Autodesk Inventor part; units mm, degrees
(part 3 of 5)
  line L1368 (280.713, 47.7132) -> (279.888, 47.7132) projected
  line L1369 (280.713, 50.3135) -> (280.713, 47.7132) projected
  line L1370 (279.888, 50.3135) -> (280.713, 50.3135) projected
  line L1371 (279.888, 53.5421) -> (279.888, 50.3135) projected
  line L1372 (273.338, 53.5421) -> (279.888, 53.5421) projected
  line L1373 (273.338, 50.3135) -> (273.338, 53.5421) projected
  line L1374 (271.614, 50.3135) -> (273.338, 50.3135) projected
  line L1375 (271.614, 55.0125) -> (271.614, 50.3135) projected
  line L1376 (226.858, 41.2129) -> (226.858, 55.0125) projected
  line L1377 (240.658, 41.2129) -> (226.858, 41.2129) projected
  line L1378 (240.658, 55.0125) -> (240.658, 41.2129) projected
  line L1379 (226.858, 55.0125) -> (240.658, 55.0125) projected
  line L1380 (221.608, 55.0125) -> (221.608, 41.2129) projected
  line L1381 (207.808, 55.0125) -> (221.608, 55.0125) projected
  line L1382 (207.808, 41.2129) -> (207.808, 55.0125) projected
  line L1383 (221.608, 41.2129) -> (207.808, 41.2129) projected
  line L1384 (202.558, 41.2129) -> (188.758, 41.2129) projected
  line L1385 (202.558, 55.0125) -> (202.558, 41.2129) projected
  line L1386 (188.758, 55.0125) -> (202.558, 55.0125) projected
  line L1387 (188.758, 41.2129) -> (188.758, 55.0125) projected
  line L1388 (122.083, 35.9625) -> (135.883, 35.9625) projected
  line L1389 (122.083, 22.163) -> (122.083, 35.9625) projected
  line L1390 (135.883, 22.163) -> (122.083, 22.163) projected
  line L1391 (135.883, 35.9625) -> (135.883, 22.163) projected
  line L1392 (195.902, 16.9127) -> (209.702, 16.9127) projected
  line L1393 (195.902, 3.113) -> (195.902, 16.9127) projected
  line L1394 (209.702, 3.113) -> (195.902, 3.113) projected
  line L1395 (209.702, 16.9127) -> (209.702, 3.113) projected
  line L1396 (193.033, 22.163) -> (179.233, 22.163) projected
  line L1397 (193.033, 35.9625) -> (193.033, 22.163) projected
  line L1398 (179.233, 35.9625) -> (193.033, 35.9625) projected
  line L1399 (179.233, 22.163) -> (179.233, 35.9625) projected
  line L1400 (160.183, 22.163) -> (160.183, 35.9625) projected
  line L1401 (173.983, 22.163) -> (160.183, 22.163) projected
  line L1402 (173.983, 35.9625) -> (173.983, 22.163) projected
  line L1403 (160.183, 35.9625) -> (173.983, 35.9625) projected
  line L1404 (141.133, 22.163) -> (141.133, 35.9625) projected
  line L1405 (154.933, 22.163) -> (141.133, 22.163) projected
  line L1406 (154.933, 35.9625) -> (154.933, 22.163) projected
  line L1407 (141.133, 35.9625) -> (154.933, 35.9625) projected
  line L1408 (73.9704, 103.125) -> (60.1694, 103.125) projected
  line L1409 (73.9704, 116.926) -> (73.9704, 103.125) projected
  line L1410 (60.1694, 116.926) -> (73.9704, 116.926) projected
  line L1411 (60.1694, 103.125) -> (60.1694, 116.926) projected
  line L1412 (131.12, 79.3129) -> (117.321, 79.3129) projected
  line L1413 (131.12, 93.1125) -> (131.12, 79.3129) projected
  line L1414 (117.321, 93.1125) -> (131.12, 93.1125) projected
  line L1415 (117.321, 79.3129) -> (117.321, 93.1125) projected
  line L1416 (112.07, 79.3129) -> (98.2694, 79.3129) projected
  line L1417 (112.07, 93.1125) -> (112.07, 79.3129) projected
  line L1418 (98.2694, 93.1125) -> (112.07, 93.1125) projected
  line L1419 (98.2694, 79.3129) -> (98.2694, 93.1125) projected
  line L1420 (140.645, 74.0625) -> (140.645, 60.2629) projected
  line L1421 (126.846, 74.0625) -> (140.645, 74.0625) projected
  line L1422 (126.846, 60.2629) -> (126.846, 74.0625) projected
  line L1423 (140.645, 60.2629) -> (126.846, 60.2629) projected
  line L1424 (145.896, 74.0625) -> (159.695, 74.0625) projected
  line L1425 (145.896, 60.2629) -> (145.896, 74.0625) projected
  line L1426 (159.695, 60.2629) -> (145.896, 60.2629) projected
  line L1427 (159.695, 74.0625) -> (159.695, 60.2629) projected
  line L1428 (93.0204, 103.125) -> (79.2194, 103.125) projected
  line L1429 (93.0204, 116.926) -> (93.0204, 103.125) projected
  line L1430 (79.2194, 116.926) -> (93.0204, 116.926) projected
  line L1431 (79.2194, 103.125) -> (79.2194, 116.926) projected
  line L1432 (112.558, 41.2129) -> (112.558, 55.0125) projected
  line L1433 (126.358, 41.2129) -> (112.558, 41.2129) projected
  line L1434 (126.358, 55.0125) -> (126.358, 41.2129) projected
  line L1435 (112.558, 55.0125) -> (126.358, 55.0125) projected
  line L1436 (54.919, 103.125) -> (41.1208, 103.125) projected
  line L1437 (54.919, 116.926) -> (54.919, 103.125) projected
  line L1438 (41.1208, 116.926) -> (54.919, 116.926) projected
  line L1439 (41.1208, 103.125) -> (41.1208, 116.926) projected
  line L1440 (102.545, 74.0625) -> (102.545, 60.2629) projected
  line L1441 (88.7444, 74.0625) -> (102.545, 74.0625) projected
  line L1442 (88.7444, 60.2629) -> (88.7444, 74.0625) projected
  line L1443 (102.545, 60.2629) -> (88.7444, 60.2629) projected
  line L1444 (107.794, 60.2629) -> (107.794, 74.0625) projected
  line L1445 (121.595, 60.2629) -> (107.794, 60.2629) projected
  line L1446 (121.595, 74.0625) -> (121.595, 60.2629) projected
  line L1447 (107.794, 74.0625) -> (121.595, 74.0625) projected
  line L1448 (79.2194, 79.3129) -> (79.2194, 93.1125) projected
  line L1449 (93.0204, 79.3129) -> (79.2194, 79.3129) projected
  line L1450 (93.0204, 93.1125) -> (93.0204, 79.3129) projected
  line L1451 (79.2194, 93.1125) -> (93.0204, 93.1125) projected
  line L1452 (73.9704, 79.3129) -> (60.1694, 79.3129) projected
  line L1453 (73.9704, 93.1125) -> (73.9704, 79.3129) projected
  line L1454 (60.1694, 93.1125) -> (73.9704, 93.1125) projected
  line L1455 (60.1694, 79.3129) -> (60.1694, 93.1125) projected
  line L1456 (50.6458, 74.0625) -> (64.4454, 74.0625) projected
  line L1457 (50.6458, 60.2629) -> (50.6458, 74.0625) projected
  line L1458 (64.4454, 60.2629) -> (50.6458, 60.2629) projected
  line L1459 (64.4454, 74.0625) -> (64.4454, 60.2629) projected
  line L1460 (83.4954, 60.2629) -> (69.6958, 60.2629) projected
  line L1461 (83.4954, 74.0625) -> (83.4954, 60.2629) projected
  line L1462 (69.6958, 74.0625) -> (83.4954, 74.0625) projected
  line L1463 (69.6958, 60.2629) -> (69.6958, 74.0625) projected
  line L1464 (74.4583, 41.2129) -> (74.4583, 55.0125) projected
  line L1465 (88.2579, 41.2129) -> (74.4583, 41.2129) projected
  line L1466 (88.2579, 55.0125) -> (88.2579, 41.2129) projected
  line L1467 (74.4583, 55.0125) -> (88.2579, 55.0125) projected
  line L1468 (41.1208, 79.3129) -> (41.1208, 93.1125) projected
  line L1469 (54.919, 79.3129) -> (41.1208, 79.3129) projected
  line L1470 (54.919, 93.1125) -> (54.919, 79.3129) projected
  line L1471 (41.1208, 93.1125) -> (54.919, 93.1125) projected
  line L1472 (107.308, 41.2129) -> (93.5083, 41.2129) projected
  line L1473 (107.308, 55.0125) -> (107.308, 41.2129) projected
  line L1474 (93.5083, 55.0125) -> (107.308, 55.0125) projected
  line L1475 (93.5083, 41.2129) -> (93.5083, 55.0125) projected
  line L1476 (103.033, 22.163) -> (103.033, 35.9625) projected
  line L1477 (116.833, 22.163) -> (103.033, 22.163) projected
  line L1478 (116.833, 35.9625) -> (116.833, 22.163) projected
  line L1479 (103.033, 35.9625) -> (116.833, 35.9625) projected
  line L1480 (97.7829, 35.9625) -> (97.7829, 22.163) projected
  line L1481 (83.9833, 35.9625) -> (97.7829, 35.9625) projected
  line L1482 (83.9833, 22.163) -> (83.9833, 35.9625) projected
  line L1483 (97.7829, 22.163) -> (83.9833, 22.163) projected
  line L1484 (16.8203, 103.125) -> (3.0193, 103.125) projected
  line L1485 (16.8203, 116.926) -> (16.8203, 103.125) projected
  line L1486 (3.0193, 116.926) -> (16.8203, 116.926) projected
  line L1487 (3.0193, 103.125) -> (3.0193, 116.926) projected
  line L1488 (16.8203, 79.3129) -> (3.0193, 79.3129) projected
  line L1489 (16.8203, 93.1125) -> (16.8203, 79.3129) projected
  line L1490 (3.0193, 93.1125) -> (16.8203, 93.1125) projected
  line L1491 (3.0193, 79.3129) -> (3.0193, 93.1125) projected
  line L1492 (35.8704, 79.3129) -> (22.0707, 79.3129) projected
  line L1493 (35.8704, 93.1125) -> (35.8704, 79.3129) projected
  line L1494 (22.0707, 93.1125) -> (35.8704, 93.1125) projected
  line L1495 (22.0707, 79.3129) -> (22.0707, 93.1125) projected
  line L1496 (31.5957, 60.2629) -> (31.5957, 74.0625) projected
  line L1497 (45.3954, 60.2629) -> (31.5957, 60.2629) projected
  line L1498 (45.3954, 74.0625) -> (45.3954, 60.2629) projected
  line L1499 (31.5957, 74.0625) -> (45.3954, 74.0625) projected
  line L1500 (21.5828, 60.2629) -> (7.7832, 60.2629) projected
  line L1501 (21.5828, 74.0625) -> (21.5828, 60.2629) projected
  line L1502 (7.7832, 74.0625) -> (21.5828, 74.0625) projected
  line L1503 (7.7832, 60.2629) -> (7.7832, 74.0625) projected
  line L1504 (50.1579, 55.0125) -> (50.1579, 41.2129) projected
  line L1505 (36.3583, 55.0125) -> (50.1579, 55.0125) projected
  line L1506 (36.3583, 41.2129) -> (36.3583, 55.0125) projected
  line L1507 (50.1579, 41.2129) -> (36.3583, 41.2129) projected
  line L1508 (69.2079, 41.2129) -> (55.4083, 41.2129) projected
  line L1509 (69.2079, 55.0125) -> (69.2079, 41.2129) projected
  line L1510 (55.4083, 55.0125) -> (69.2079, 55.0125) projected
  line L1511 (55.4083, 41.2129) -> (55.4083, 55.0125) projected
  line L1512 (78.7329, 22.163) -> (64.9333, 22.163) projected
  line L1513 (78.7329, 35.9625) -> (78.7329, 22.163) projected
  line L1514 (64.9333, 35.9625) -> (78.7329, 35.9625) projected
  line L1515 (64.9333, 22.163) -> (64.9333, 35.9625) projected
  line L1516 (53.0271, 16.9127) -> (66.8267, 16.9127) projected
  line L1517 (53.0271, 3.113) -> (53.0271, 16.9127) projected
  line L1518 (66.8267, 3.113) -> (53.0271, 3.113) projected
  line L1519 (66.8267, 16.9127) -> (66.8267, 3.113) projected
  line L1520 (78.0881, 15.4423) -> (84.6391, 15.4423) projected
  line L1521 (78.0881, 12.2136) -> (78.0881, 15.4423) projected
  line L1522 (77.264, 12.2136) -> (78.0881, 12.2136) projected
  line L1523 (77.264, 9.6132) -> (77.264, 12.2136) projected
  line L1524 (78.0881, 9.6132) -> (77.264, 9.6132) projected
  line L1525 (78.0881, 3.3431) -> (78.0881, 9.6132) projected
  line L1526 (79.8132, 3.3431) -> (78.0881, 3.3431) projected
  line L1527 (79.8132, 2.1429) -> (79.8132, 3.3431) projected
  line L1528 (82.9137, 2.1429) -> (79.8132, 2.1429) projected
  line L1529 (82.9137, 3.3431) -> (82.9137, 2.1429) projected
  line L1530 (84.6391, 3.3431) -> (82.9137, 3.3431) projected
  line L1531 (84.6391, 7.8135) -> (84.6391, 3.3431) projected
  line L1532 (124.463, 7.8135) -> (84.6391, 7.8135) projected
  line L1533 (124.463, 3.113) -> (124.463, 7.8135) projected
  line L1534 (138.264, 3.113) -> (124.463, 3.113) projected
  line L1535 (138.264, 7.8135) -> (138.264, 3.113) projected
  line L1536 (178.088, 7.8135) -> (138.264, 7.8135) projected
  line L1537 (178.088, 3.3431) -> (178.088, 7.8135) projected
  line L1538 (179.813, 3.3431) -> (178.088, 3.3431) projected
  line L1539 (179.813, 2.1429) -> (179.813, 3.3431) projected
  line L1540 (182.914, 2.1429) -> (179.813, 2.1429) projected
  line L1541 (182.914, 3.3431) -> (182.914, 2.1429) projected
  line L1542 (184.638, 3.3431) -> (182.914, 3.3431) projected
  line L1543 (184.638, 9.6132) -> (184.638, 3.3431) projected
  line L1544 (185.463, 9.6132) -> (184.638, 9.6132) projected
  line L1545 (185.463, 12.2136) -> (185.463, 9.6132) projected
  line L1546 (184.638, 12.2136) -> (185.463, 12.2136) projected
  line L1547 (184.638, 15.4423) -> (184.638, 12.2136) projected
  line L1548 (178.088, 15.4423) -> (184.638, 15.4423) projected
  line L1549 (178.088, 12.2136) -> (178.088, 15.4423) projected
  line L1550 (138.264, 12.2136) -> (178.088, 12.2136) projected
  line L1551 (138.264, 16.9127) -> (138.264, 12.2136) projected
  line L1552 (124.463, 16.9127) -> (138.264, 16.9127) projected
  line L1553 (124.463, 12.2136) -> (124.463, 16.9127) projected
  line L1554 (84.6391, 12.2136) -> (124.463, 12.2136) projected
  line L1555 (84.6391, 15.4423) -> (84.6391, 12.2136) projected
  line L1556 (23.9641, 55.0125) -> (23.9641, 41.2129) projected
  line L1557 (10.163, 55.0125) -> (23.9641, 55.0125) projected
  line L1558 (10.163, 41.2129) -> (10.163, 55.0125) projected
  line L1559 (23.9641, 41.2129) -> (10.163, 41.2129) projected
  line L1560 (28.7266, 35.9625) -> (28.7266, 31.2636) projected
  line L1561 (14.9269, 35.9625) -> (28.7266, 35.9625) projected
  line L1562 (14.9269, 31.2636) -> (14.9269, 35.9625) projected
  line L1563 (13.2016, 31.2636) -> (14.9269, 31.2636) projected
  line L1564 (13.2016, 34.4923) -> (13.2016, 31.2636) projected
  line L1565 (6.6518, 34.4923) -> (13.2016, 34.4923) projected
  line L1566 (6.6518, 31.2636) -> (6.6518, 34.4923) projected
  line L1567 (5.8263, 31.2636) -> (6.6518, 31.2636) projected
  line L1568 (5.8263, 28.6632) -> (5.8263, 31.2636) projected
  line L1569 (6.6518, 28.6632) -> (5.8263, 28.6632) projected
  line L1570 (6.6518, 22.3931) -> (6.6518, 28.6632) projected
  line L1571 (8.3771, 22.3931) -> (6.6518, 22.3931) projected
  line L1572 (8.3771, 21.1928) -> (8.3771, 22.3931) projected
  line L1573 (11.4763, 21.1928) -> (8.3771, 21.1928) projected
  line L1574 (11.4763, 22.3931) -> (11.4763, 21.1928) projected
  line L1575 (13.2016, 22.3931) -> (11.4763, 22.3931) projected
  line L1576 (13.2016, 26.8635) -> (13.2016, 22.3931) projected
  line L1577 (14.9269, 26.8635) -> (13.2016, 26.8635) projected
  line L1578 (14.9269, 22.163) -> (14.9269, 26.8635) projected
  line L1579 (28.7266, 22.163) -> (14.9269, 22.163) projected
  line L1580 (28.7266, 26.8635) -> (28.7266, 22.163) projected
  line L1581 (30.4519, 26.8635) -> (28.7266, 26.8635) projected
  line L1582 (30.4519, 22.3931) -> (30.4519, 26.8635) projected
  line L1583 (32.1758, 22.3931) -> (30.4519, 22.3931) projected
  line L1584 (32.1758, 21.1928) -> (32.1758, 22.3931) projected
  line L1585 (35.2764, 21.1928) -> (32.1758, 21.1928) projected
  line L1586 (35.2764, 22.3931) -> (35.2764, 21.1928) projected
  line L1587 (37.0018, 22.3931) -> (35.2764, 22.3931) projected
  line L1588 (37.0018, 28.6632) -> (37.0018, 22.3931) projected
  line L1589 (37.8273, 28.6632) -> (37.0018, 28.6632) projected
  line L1590 (37.8273, 31.2636) -> (37.8273, 28.6632) projected
  line L1591 (37.0018, 31.2636) -> (37.8273, 31.2636) projected
  line L1592 (37.0018, 34.4923) -> (37.0018, 31.2636) projected
  line L1593 (30.4519, 34.4923) -> (37.0018, 34.4923) projected
  line L1594 (30.4519, 31.2636) -> (30.4519, 34.4923) projected
  line L1595 (28.7266, 31.2636) -> (30.4519, 31.2636) projected
  line L1596 (98.2694, 116.926) -> (112.07, 116.926) projected
  line L1597 (98.2694, 103.125) -> (98.2694, 116.926) projected
  line L1598 (112.07, 103.125) -> (98.2694, 103.125) projected
  line L1599 (112.07, 116.926) -> (112.07, 103.125) projected
  line L1600 (135.883, 116.926) -> (135.883, 103.125) projected
  line L1601 (122.083, 116.926) -> (135.883, 116.926) projected
  line L1602 (122.083, 103.125) -> (122.083, 116.926) projected
  line L1603 (135.883, 103.125) -> (122.083, 103.125) projected
  line L1604 (2.096, 0.1874) -> (303.496, 0.1874) projected
  line L1605 (2.096, 0.1874) -> (303.496, 0.1874) projected
  line L1606 (2.096, 0.1874) -> (303.496, 0.1874) projected
  line L1607 (2.096, 0.1874) -> (303.496, 0.1874) projected
  line L1608 (145.408, 41.2129) -> (131.608, 41.2129) projected
  line L1609 (198.283, 35.9625) -> (212.083, 35.9625) projected
  line L1610 (198.283, 35.9625) -> (212.083, 35.9625) projected
  line L1611 (207.808, 55.0125) -> (221.608, 55.0125) projected
  line L1612 (221.608, 41.2129) -> (207.808, 41.2129) projected
  line L1613 (221.608, 41.2129) -> (207.808, 41.2129) projected
  line L1614 (221.608, 55.0125) -> (221.608, 41.2129) projected
  line L1615 (241.146, 60.2629) -> (241.146, 74.0625) projected
  line L1616 (212.571, 93.1125) -> (226.37, 93.1125) projected
  line L1617 (0.9192, 119.469) -> (0.7965, 119.371) projected
  line L1618 (145.408, 41.2129) -> (131.608, 41.2129) projected
  line L1619 (212.571, 79.3129) -> (212.571, 93.1125) projected
  line L1620 (221.608, 55.0125) -> (221.608, 41.2129) projected
  line L1621 (0.39, 118.894) -> (0.3128, 118.758) projected
  line L1622 (0.39, 118.894) -> (0.3128, 118.758) projected
  line L1623 (0.3128, 118.758) -> (0.248, 118.616) projected
  line L1624 (0.3128, 118.758) -> (0.248, 118.616) projected
  line L1625 (0.248, 118.616) -> (0.1929, 118.468) projected
  line L1626 (0.248, 118.616) -> (0.1929, 118.468) projected
  line L1627 (0.1929, 118.468) -> (0.1502, 118.317) projected
  line L1628 (226.37, 79.3129) -> (212.571, 79.3129) projected
  line L1629 (145.408, 55.0125) -> (145.408, 41.2129) projected
  line L1630 (0.1199, 118.163) -> (0.102, 118.007) projected
  line L1631 (0.1199, 118.163) -> (0.102, 118.007) projected
  line L1632 (0.1502, 118.317) -> (0.1199, 118.163) projected
  line L1633 (0.1502, 118.317) -> (0.1199, 118.163) projected
  line L1634 (0.1929, 118.468) -> (0.1502, 118.317) projected
  line L1635 (0.102, 118.007) -> (0.0951, 117.85) projected
  line L1636 (0.102, 118.007) -> (0.0951, 117.85) projected
  line L1637 (0.0951, 117.85) -> (0.0951, 2.187) projected
  line L1638 (0.0951, 117.85) -> (0.0951, 2.187) projected
  line L1639 (0.0951, 2.187) -> (0.102, 2.0298) projected
  line L1640 (0.0951, 2.187) -> (0.102, 2.0298) projected
  line L1641 (0.102, 2.0298) -> (0.1199, 1.8741) projected
  line L1642 (0.102, 2.0298) -> (0.1199, 1.8741) projected
  line L1643 (0.1199, 1.8741) -> (0.1502, 1.7198) projected
  line L1644 (0.1199, 1.8741) -> (0.1502, 1.7198) projected
  line L1645 (0.1502, 1.7198) -> (0.1929, 1.5696) projected
  line L1646 (0.1929, 1.5696) -> (0.248, 1.4221) projected
  line L1647 (0.1502, 1.7198) -> (0.1929, 1.5696) projected
  line L1648 (0.39, 1.1424) -> (0.4768, 1.0115) projected
  line L1649 (0.3128, 1.2788) -> (0.39, 1.1424) projected
  line L1650 (0.248, 1.4221) -> (0.3128, 1.2788) projected
  line L1651 (0.248, 1.4221) -> (0.3128, 1.2788) projected
  line L1652 (0.1929, 1.5696) -> (0.248, 1.4221) projected
  line L1653 (0.3128, 1.2788) -> (0.39, 1.1424) projected
  line L1654 (0.6808, 0.7731) -> (0.7965, 0.6656) projected
  line L1655 (0.5746, 0.8875) -> (0.6808, 0.7731) projected
  line L1656 (0.5746, 0.8875) -> (0.6808, 0.7731) projected
  line L1657 (0.4768, 1.0115) -> (0.5746, 0.8875) projected
  line L1658 (0.4768, 1.0115) -> (0.5746, 0.8875) projected
  line L1659 (0.39, 1.1424) -> (0.4768, 1.0115) projected
  line L1660 (1.0501, 0.4823) -> (1.1879, 0.4051) projected
  line L1661 (0.9192, 0.5691) -> (1.0501, 0.4823) projected
  line L1662 (0.9192, 0.5691) -> (1.0501, 0.4823) projected
  line L1663 (0.7965, 0.6656) -> (0.9192, 0.5691) projected
  line L1664 (0.6808, 0.7731) -> (0.7965, 0.6656) projected
  line L1665 (0.7965, 0.6656) -> (0.9192, 0.5691) projected
  line L1666 (1.4759, 0.2853) -> (1.6288, 0.2425) projected
  line L1667 (1.3298, 0.339) -> (1.4759, 0.2853) projected
  line L1668 (1.3298, 0.339) -> (1.4759, 0.2853) projected
  line L1669 (1.1879, 0.4051) -> (1.3298, 0.339) projected
  line L1670 (1.0501, 0.4823) -> (1.1879, 0.4051) projected
  line L1671 (1.1879, 0.4051) -> (1.3298, 0.339) projected
  line L1672 (1.9389, 0.1929) -> (2.096, 0.1874) projected
  line L1673 (1.9389, 0.1929) -> (2.096, 0.1874) projected
  line L1674 (1.7818, 0.2122) -> (1.9389, 0.1929) projected
  line L1675 (1.7818, 0.2122) -> (1.9389, 0.1929) projected
  line L1676 (1.6288, 0.2425) -> (1.7818, 0.2122) projected
  line L1677 (1.4759, 0.2853) -> (1.6288, 0.2425) projected
  line L1678 (1.6288, 0.2425) -> (1.7818, 0.2122) projected
  line L1679 (145.408, 55.0125) -> (145.408, 41.2129) projected
  line L1680 (59.6829, 35.9625) -> (59.6829, 22.163) projected
  line L1681 (59.6829, 35.9625) -> (59.6829, 22.163) projected
  line L1682 (59.6829, 22.163) -> (45.8833, 22.163) projected
  line L1683 (59.6829, 22.163) -> (45.8833, 22.163) projected
  line L1684 (45.8833, 22.163) -> (45.8833, 35.9625) projected
  line L1685 (45.8833, 22.163) -> (45.8833, 35.9625) projected
  line L1686 (212.571, 93.1125) -> (226.37, 93.1125) projected
  line L1687 (150.658, 55.0125) -> (164.458, 55.0125) projected
  line L1688 (150.658, 55.0125) -> (164.458, 55.0125) projected
  line L1689 (164.458, 41.2129) -> (150.658, 41.2129) projected
  line L1690 (164.458, 41.2129) -> (150.658, 41.2129) projected
  line L1691 (150.658, 41.2129) -> (150.658, 55.0125) projected
  line L1692 (150.658, 41.2129) -> (150.658, 55.0125) projected
  line L1693 (131.608, 55.0125) -> (145.408, 55.0125) projected
  line L1694 (131.608, 41.2129) -> (131.608, 55.0125) projected
  line L1695 (131.608, 41.2129) -> (131.608, 55.0125) projected
  line L1696 (131.608, 55.0125) -> (145.408, 55.0125) projected
  line L1697 (45.8833, 35.9625) -> (59.6829, 35.9625) projected
  line L1698 (19.2016, 16.9127) -> (19.2016, 3.113) projected
  line L1699 (19.2016, 16.9127) -> (19.2016, 3.113) projected
  line L1700 (5.4019, 16.9127) -> (19.2016, 16.9127) projected
  line L1701 (5.4019, 16.9127) -> (19.2016, 16.9127) projected
  line L1702 (45.8833, 35.9625) -> (59.6829, 35.9625) projected
  line L1703 (29.213, 16.9127) -> (43.0142, 16.9127) projected
  line L1704 (29.213, 16.9127) -> (43.0142, 16.9127) projected
  line L1705 (5.4019, 3.113) -> (5.4019, 16.9127) projected
  line L1706 (5.4019, 3.113) -> (5.4019, 16.9127) projected
  line L1707 (19.2016, 3.113) -> (5.4019, 3.113) projected
  line L1708 (183.508, 55.0125) -> (183.508, 41.2129) projected
  line L1709 (183.508, 55.0125) -> (183.508, 41.2129) projected
  line L1710 (183.508, 41.2129) -> (169.708, 41.2129) projected
  line L1711 (183.508, 41.2129) -> (169.708, 41.2129) projected
  line L1712 (169.708, 41.2129) -> (169.708, 55.0125) projected
  line L1713 (169.708, 41.2129) -> (169.708, 55.0125) projected
  line L1714 (164.458, 55.0125) -> (164.458, 41.2129) projected
  line L1715 (164.458, 55.0125) -> (164.458, 41.2129) projected
  line L1716 (226.37, 93.1125) -> (226.37, 79.3129) projected
  line L1717 (222.096, 116.926) -> (235.895, 116.926) projected
  line L1718 (222.096, 103.125) -> (222.096, 116.926) projected
  line L1719 (212.571, 79.3129) -> (212.571, 93.1125) projected
  line L1720 (188.27, 93.1125) -> (188.27, 79.3129) projected
  line L1721 (174.471, 93.1125) -> (188.27, 93.1125) projected
  line L1722 (169.708, 55.0125) -> (183.508, 55.0125) projected
  line L1723 (222.096, 116.926) -> (235.895, 116.926) projected
  line L1724 (212.083, 35.9625) -> (212.083, 22.163) projected
  line L1725 (212.083, 35.9625) -> (212.083, 22.163) projected
  line L1726 (198.283, 22.163) -> (198.283, 35.9625) projected
  line L1727 (212.083, 22.163) -> (198.283, 22.163) projected
  line L1728 (198.283, 22.163) -> (198.283, 35.9625) projected
  line L1729 (207.808, 41.2129) -> (207.808, 55.0125) projected
  line L1730 (43.0142, 16.9127) -> (43.0142, 3.113) projected
  line L1731 (43.0142, 3.113) -> (29.213, 3.113) projected
  line L1732 (29.213, 3.113) -> (29.213, 16.9127) projected
  line L1733 (43.0142, 3.113) -> (29.213, 3.113) projected
  line L1734 (29.213, 3.113) -> (29.213, 16.9127) projected
  line L1735 (43.0142, 16.9127) -> (43.0142, 3.113) projected
  line L1736 (19.2016, 3.113) -> (5.4019, 3.113) projected
  line L1737 (251.92, 88.4135) -> (251.92, 91.6421) projected
  line L1738 (174.471, 79.3129) -> (174.471, 93.1125) projected
  line L1739 (174.471, 79.3129) -> (174.471, 93.1125) projected
  line L1740 (188.27, 93.1125) -> (188.27, 79.3129) projected
  line L1741 (212.571, 93.1125) -> (226.37, 93.1125) projected
  line L1742 (212.571, 93.1125) -> (226.37, 93.1125) projected
  line L1743 (226.37, 79.3129) -> (212.571, 79.3129) projected
  line L1744 (226.37, 79.3129) -> (212.571, 79.3129) projected
  line L1745 (226.37, 93.1125) -> (226.37, 79.3129) projected
  line L1746 (226.37, 93.1125) -> (226.37, 79.3129) projected
  line L1747 (212.571, 79.3129) -> (212.571, 93.1125) projected
  line L1748 (212.571, 79.3129) -> (212.571, 93.1125) projected
  line L1749 (193.521, 93.1125) -> (207.32, 93.1125) projected
  line L1750 (193.521, 93.1125) -> (207.32, 93.1125) projected
  line L1751 (193.521, 93.1125) -> (207.32, 93.1125) projected
  line L1752 (207.32, 93.1125) -> (207.32, 79.3129) projected
  line L1753 (207.32, 93.1125) -> (207.32, 79.3129) projected
  line L1754 (207.32, 93.1125) -> (207.32, 79.3129) projected
  line L1755 (207.32, 93.1125) -> (207.32, 79.3129) projected
  line L1756 (207.32, 79.3129) -> (193.521, 79.3129) projected
  line L1757 (193.521, 79.3129) -> (193.521, 93.1125) projected
  line L1758 (193.521, 79.3129) -> (193.521, 93.1125) projected
  line L1759 (193.521, 79.3129) -> (193.521, 93.1125) projected
  line L1760 (207.32, 79.3129) -> (193.521, 79.3129) projected
  line L1761 (207.32, 79.3129) -> (193.521, 79.3129) projected
  line L1762 (207.32, 79.3129) -> (193.521, 79.3129) projected
  line L1763 (193.521, 79.3129) -> (193.521, 93.1125) projected
  line L1764 (193.521, 93.1125) -> (207.32, 93.1125) projected
  line L1765 (216.845, 60.2629) -> (203.046, 60.2629) projected
  line L1766 (216.845, 60.2629) -> (203.046, 60.2629) projected
  line L1767 (216.845, 60.2629) -> (203.046, 60.2629) projected
  line L1768 (216.845, 60.2629) -> (203.046, 60.2629) projected
  line L1769 (202.558, 55.0125) -> (202.558, 41.2129) projected
  line L1770 (202.558, 55.0125) -> (202.558, 41.2129) projected
  line L1771 (202.558, 41.2129) -> (188.758, 41.2129) projected
  line L1772 (202.558, 41.2129) -> (188.758, 41.2129) projected
  line L1773 (188.758, 41.2129) -> (188.758, 55.0125) projected
  line L1774 (188.758, 41.2129) -> (188.758, 55.0125) projected
  line L1775 (188.758, 55.0125) -> (202.558, 55.0125) projected
  line L1776 (188.758, 55.0125) -> (202.558, 55.0125) projected
  line L1777 (216.845, 74.0625) -> (216.845, 60.2629) projected
  line L1778 (216.845, 74.0625) -> (216.845, 60.2629) projected
  line L1779 (216.845, 74.0625) -> (216.845, 60.2629) projected
  line L1780 (216.845, 74.0625) -> (216.845, 60.2629) projected
  line L1781 (203.046, 60.2629) -> (203.046, 74.0625) projected
  line L1782 (203.046, 60.2629) -> (203.046, 74.0625) projected
  line L1783 (203.046, 60.2629) -> (203.046, 74.0625) projected
  line L1784 (203.046, 60.2629) -> (203.046, 74.0625) projected
  line L1785 (203.046, 74.0625) -> (216.845, 74.0625) projected
  line L1786 (203.046, 74.0625) -> (216.845, 74.0625) projected
  line L1787 (203.046, 74.0625) -> (216.845, 74.0625) projected
  line L1788 (203.046, 74.0625) -> (216.845, 74.0625) projected
  line L1789 (251.095, 85.8132) -> (251.095, 88.4135) projected
  line L1790 (248.714, 47.7132) -> (248.714, 50.3135) projected
  line L1791 (240.658, 55.0125) -> (240.658, 41.2129) projected
  line L1792 (226.858, 55.0125) -> (240.658, 55.0125) projected
  line L1793 (226.858, 55.0125) -> (240.658, 55.0125) projected
  line L1794 (226.858, 41.2129) -> (226.858, 55.0125) projected
  line L1795 (226.858, 41.2129) -> (226.858, 55.0125) projected
  line L1796 (240.658, 41.2129) -> (226.858, 41.2129) projected
  line L1797 (240.658, 41.2129) -> (226.858, 41.2129) projected
  line L1798 (248.714, 47.7132) -> (248.714, 50.3135) projected
  line L1799 (193.033, 116.926) -> (193.033, 103.125) projected
  line L1800 (193.033, 116.926) -> (193.033, 103.125) projected
  line L1801 (216.845, 103.125) -> (203.046, 103.125) projected
  line L1802 (216.845, 103.125) -> (203.046, 103.125) projected
  line L1803 (203.046, 103.125) -> (203.046, 116.926) projected
  line L1804 (203.046, 103.125) -> (203.046, 116.926) projected
  line L1805 (203.046, 116.926) -> (216.845, 116.926) projected
  line L1806 (203.046, 116.926) -> (216.845, 116.926) projected
  line L1807 (193.033, 116.926) -> (193.033, 103.125) projected
  line L1808 (193.033, 116.926) -> (193.033, 103.125) projected
  line L1809 (216.845, 103.125) -> (203.046, 103.125) projected
  line L1810 (216.845, 103.125) -> (203.046, 103.125) projected
  line L1811 (203.046, 103.125) -> (203.046, 116.926) projected
  line L1812 (203.046, 103.125) -> (203.046, 116.926) projected
  line L1813 (216.845, 116.926) -> (216.845, 103.125) projected
  line L1814 (216.845, 116.926) -> (216.845, 103.125) projected
  line L1815 (216.845, 116.926) -> (216.845, 103.125) projected
  line L1816 (216.845, 116.926) -> (216.845, 103.125) projected
  line L1817 (222.096, 103.125) -> (222.096, 116.926) projected
  line L1818 (222.096, 103.125) -> (222.096, 116.926) projected
  line L1819 (235.895, 103.125) -> (222.096, 103.125) projected
  line L1820 (235.895, 103.125) -> (222.096, 103.125) projected
  line L1821 (235.895, 116.926) -> (235.895, 103.125) projected
  line L1822 (235.895, 116.926) -> (235.895, 103.125) projected
  line L1823 (222.096, 116.926) -> (235.895, 116.926) projected
  line L1824 (222.096, 116.926) -> (235.895, 116.926) projected
  line L1825 (203.046, 116.926) -> (216.845, 116.926) projected
  line L1826 (203.046, 116.926) -> (216.845, 116.926) projected
  line L1827 (188.27, 79.3129) -> (174.471, 79.3129) projected
  line L1828 (188.27, 79.3129) -> (174.471, 79.3129) projected
  line L1829 (207.808, 41.2129) -> (207.808, 55.0125) projected
  line L1830 (235.895, 60.2629) -> (222.096, 60.2629) projected
  line L1831 (235.895, 60.2629) -> (222.096, 60.2629) projected
  line L1832 (222.096, 60.2629) -> (222.096, 74.0625) projected
  line L1833 (222.096, 60.2629) -> (222.096, 74.0625) projected
  line L1834 (222.096, 74.0625) -> (235.895, 74.0625) projected
  line L1835 (222.096, 74.0625) -> (235.895, 74.0625) projected
  line L1836 (235.895, 74.0625) -> (235.895, 60.2629) projected
  line L1837 (235.895, 74.0625) -> (235.895, 60.2629) projected
  line L1838 (207.808, 55.0125) -> (221.608, 55.0125) projected
  line L1839 (207.808, 55.0125) -> (221.608, 55.0125) projected
  line L1840 (222.096, 60.2629) -> (222.096, 74.0625) projected
  line L1841 (222.096, 60.2629) -> (222.096, 74.0625) projected
  line L1842 (222.096, 74.0625) -> (235.895, 74.0625) projected
  line L1843 (222.096, 74.0625) -> (235.895, 74.0625) projected
  line L1844 (235.895, 74.0625) -> (235.895, 60.2629) projected
  line L1845 (235.895, 74.0625) -> (235.895, 60.2629) projected
  line L1846 (241.146, 60.2629) -> (241.146, 74.0625) projected
  line L1847 (241.146, 60.2629) -> (241.146, 74.0625) projected
  line L1848 (235.895, 60.2629) -> (222.096, 60.2629) projected
  line L1849 (235.895, 60.2629) -> (222.096, 60.2629) projected
  line L1850 (207.808, 41.2129) -> (207.808, 55.0125) projected
  line L1851 (207.808, 41.2129) -> (207.808, 55.0125) projected
  line L1852 (221.608, 55.0125) -> (221.608, 41.2129) projected
  line L1853 (221.608, 55.0125) -> (221.608, 41.2129) projected
  line L1854 (226.858, 41.2129) -> (226.858, 55.0125) projected
  line L1855 (226.858, 41.2129) -> (226.858, 55.0125) projected
  line L1856 (226.858, 55.0125) -> (240.658, 55.0125) projected
  line L1857 (226.858, 55.0125) -> (240.658, 55.0125) projected
  line L1858 (240.658, 55.0125) -> (240.658, 41.2129) projected
  line L1859 (240.658, 55.0125) -> (240.658, 41.2129) projected
  line L1860 (240.658, 41.2129) -> (226.858, 41.2129) projected
  line L1861 (240.658, 41.2129) -> (226.858, 41.2129) projected
  line L1862 (221.608, 41.2129) -> (207.808, 41.2129) projected
  line L1863 (221.608, 41.2129) -> (207.808, 41.2129) projected
  line L1864 (183.996, 74.0625) -> (197.795, 74.0625) projected
  line L1865 (183.996, 74.0625) -> (197.795, 74.0625) projected
  line L1866 (183.996, 74.0625) -> (197.795, 74.0625) projected
  line L1867 (183.996, 74.0625) -> (197.795, 74.0625) projected
  line L1868 (197.795, 74.0625) -> (197.795, 60.2629) projected
  line L1869 (197.795, 74.0625) -> (197.795, 60.2629) projected
  line L1870 (197.795, 74.0625) -> (197.795, 60.2629) projected
  line L1871 (197.795, 74.0625) -> (197.795, 60.2629) projected
  line L1872 (197.795, 60.2629) -> (183.996, 60.2629) projected
  line L1873 (197.795, 60.2629) -> (183.996, 60.2629) projected
  line L1874 (197.795, 60.2629) -> (183.996, 60.2629) projected
  line L1875 (197.795, 60.2629) -> (183.996, 60.2629) projected
  line L1876 (183.996, 60.2629) -> (183.996, 74.0625) projected
  line L1877 (183.996, 60.2629) -> (183.996, 74.0625) projected
  line L1878 (183.996, 60.2629) -> (183.996, 74.0625) projected
  line L1879 (183.996, 60.2629) -> (183.996, 74.0625) projected
  line L1880 (193.033, 103.125) -> (179.233, 103.125) projected
  line L1881 (193.033, 103.125) -> (179.233, 103.125) projected
  line L1882 (179.233, 103.125) -> (179.233, 116.926) projected
  line L1883 (179.233, 103.125) -> (179.233, 116.926) projected
  line L1884 (179.233, 116.926) -> (193.033, 116.926) projected
  line L1885 (179.233, 116.926) -> (193.033, 116.926) projected
  line L1886 (174.471, 93.1125) -> (188.27, 93.1125) projected
  line L1887 (178.745, 74.0625) -> (178.745, 60.2629) projected
  line L1888 (178.745, 74.0625) -> (178.745, 60.2629) projected
  line L1889 (178.745, 60.2629) -> (164.946, 60.2629) projected
  line L1890 (178.745, 60.2629) -> (164.946, 60.2629) projected
  line L1891 (164.946, 74.0625) -> (178.745, 74.0625) projected
  line L1892 (164.946, 74.0625) -> (178.745, 74.0625) projected
  line L1893 (164.946, 60.2629) -> (164.946, 74.0625) projected
  line L1894 (164.946, 60.2629) -> (164.946, 74.0625) projected
  line L1895 (251.095, 85.8132) -> (251.095, 88.4135) projected
  line L1896 (173.983, 103.125) -> (160.183, 103.125) projected
  line L1897 (173.983, 103.125) -> (160.183, 103.125) projected
  line L1898 (173.983, 116.926) -> (173.983, 103.125) projected
  line L1899 (173.983, 116.926) -> (173.983, 103.125) projected
  line L1900 (160.183, 103.125) -> (160.183, 116.926) projected
  line L1901 (160.183, 116.926) -> (173.983, 116.926) projected
  line L1902 (160.183, 116.926) -> (173.983, 116.926) projected
  line L1903 (154.933, 103.125) -> (141.133, 103.125) projected
  line L1904 (154.933, 103.125) -> (141.133, 103.125) projected
  line L1905 (141.133, 103.125) -> (141.133, 116.926) projected
  line L1906 (141.133, 103.125) -> (141.133, 116.926) projected
  line L1907 (141.133, 116.926) -> (154.933, 116.926) projected
  line L1908 (141.133, 116.926) -> (154.933, 116.926) projected
  line L1909 (154.933, 116.926) -> (154.933, 103.125) projected
  line L1910 (154.933, 116.926) -> (154.933, 103.125) projected
  line L1911 (160.183, 103.125) -> (160.183, 116.926) projected
  line L1912 (150.17, 93.1125) -> (150.17, 79.3129) projected
  line L1913 (150.17, 93.1125) -> (150.17, 79.3129) projected
  line L1914 (150.17, 79.3129) -> (136.371, 79.3129) projected
  line L1915 (150.17, 79.3129) -> (136.371, 79.3129) projected
  line L1916 (136.371, 79.3129) -> (136.371, 93.1125) projected
  line L1917 (136.371, 79.3129) -> (136.371, 93.1125) projected
  line L1918 (136.371, 93.1125) -> (150.17, 93.1125) projected
  line L1919 (136.371, 93.1125) -> (150.17, 93.1125) projected
  line L1920 (169.22, 79.3129) -> (155.421, 79.3129) projected
  line L1921 (169.22, 79.3129) -> (155.421, 79.3129) projected
  line L1922 (155.421, 79.3129) -> (155.421, 93.1125) projected
  line L1923 (169.22, 93.1125) -> (169.22, 79.3129) projected
  line L1924 (169.22, 93.1125) -> (169.22, 79.3129) projected
  line L1925 (155.421, 93.1125) -> (169.22, 93.1125) projected
  line L1926 (155.421, 93.1125) -> (169.22, 93.1125) projected
  line L1927 (155.421, 79.3129) -> (155.421, 93.1125) projected
  line L1928 (169.708, 55.0125) -> (183.508, 55.0125) projected
  line L1929 (212.083, 22.163) -> (198.283, 22.163) projected
  line L1930 (202.558, 55.0125) -> (202.558, 41.2129) projected
  line L1931 (202.558, 55.0125) -> (202.558, 41.2129) projected
  line L1932 (188.758, 41.2129) -> (188.758, 55.0125) projected
  line L1933 (188.758, 55.0125) -> (202.558, 55.0125) projected
  line L1934 (207.808, 55.0125) -> (221.608, 55.0125) projected
  line L1935 (209.702, 16.9127) -> (209.702, 3.113) projected
  line L1936 (209.702, 3.113) -> (195.902, 3.113) projected
  line L1937 (195.902, 3.113) -> (195.902, 16.9127) projected
  line L1938 (195.902, 3.113) -> (195.902, 16.9127) projected
  line L1939 (188.758, 55.0125) -> (202.558, 55.0125) projected
  line L1940 (188.758, 41.2129) -> (188.758, 55.0125) projected
  line L1941 (219.713, 16.9127) -> (233.514, 16.9127) projected
  line L1942 (219.713, 16.9127) -> (233.514, 16.9127) projected
  line L1943 (233.514, 16.9127) -> (233.514, 3.113) projected
  line L1944 (233.514, 16.9127) -> (233.514, 3.113) projected
  line L1945 (233.514, 3.113) -> (219.713, 3.113) projected
  line L1946 (233.514, 3.113) -> (219.713, 3.113) projected
  line L1947 (219.713, 3.113) -> (219.713, 16.9127) projected
  line L1948 (219.713, 3.113) -> (219.713, 16.9127) projected
  line L1949 (217.333, 35.9625) -> (231.133, 35.9625) projected
  line L1950 (217.333, 35.9625) -> (231.133, 35.9625) projected
  line L1951 (231.133, 35.9625) -> (231.133, 22.163) projected
  line L1952 (231.133, 35.9625) -> (231.133, 22.163) projected
  line L1953 (231.133, 22.163) -> (217.333, 22.163) projected
  line L1954 (231.133, 22.163) -> (217.333, 22.163) projected
  line L1955 (217.333, 22.163) -> (217.333, 35.9625) projected
  line L1956 (217.333, 22.163) -> (217.333, 35.9625) projected
  line L1957 (198.283, 35.9625) -> (212.083, 35.9625) projected
  line L1958 (198.283, 35.9625) -> (212.083, 35.9625) projected
  line L1959 (212.083, 35.9625) -> (212.083, 22.163) projected
  line L1960 (212.083, 35.9625) -> (212.083, 22.163) projected
  line L1961 (212.083, 22.163) -> (198.283, 22.163) projected
  line L1962 (212.083, 22.163) -> (198.283, 22.163) projected
  line L1963 (198.283, 22.163) -> (198.283, 35.9625) projected
  line L1964 (198.283, 22.163) -> (198.283, 35.9625) projected
  line L1965 (195.902, 16.9127) -> (209.702, 16.9127) projected
  line L1966 (195.902, 16.9127) -> (209.702, 16.9127) projected
  line L1967 (179.233, 35.9625) -> (193.033, 35.9625) projected
  line L1968 (179.233, 35.9625) -> (193.033, 35.9625) projected
  line L1969 (209.702, 16.9127) -> (209.702, 3.113) projected
  line L1970 (209.702, 16.9127) -> (209.702, 3.113) projected
  line L1971 (209.702, 3.113) -> (195.902, 3.113) projected
  line L1972 (209.702, 3.113) -> (195.902, 3.113) projected
  line L1973 (184.638, 15.4423) -> (184.638, 12.2136) projected
  line L1974 (184.638, 15.4423) -> (184.638, 12.2136) projected
  line L1975 (184.638, 12.2136) -> (185.463, 12.2136) projected
  line L1976 (184.638, 12.2136) -> (185.463, 12.2136) projected
  line L1977 (179.233, 22.163) -> (179.233, 35.9625) projected
  line L1978 (179.233, 22.163) -> (179.233, 35.9625) projected
  line L1979 (193.033, 22.163) -> (179.233, 22.163) projected
  line L1980 (193.033, 22.163) -> (179.233, 22.163) projected
  line L1981 (185.463, 12.2136) -> (185.463, 9.6132) projected
  line L1982 (185.463, 12.2136) -> (185.463, 9.6132) projected
  line L1983 (195.902, 3.113) -> (195.902, 16.9127) projected
  line L1984 (195.902, 3.113) -> (195.902, 16.9127) projected
  line L1985 (185.463, 9.6132) -> (184.638, 9.6132) projected
  line L1986 (185.463, 9.6132) -> (184.638, 9.6132) projected
  line L1987 (178.088, 15.4423) -> (184.638, 15.4423) projected
  line L1988 (178.088, 15.4423) -> (184.638, 15.4423) projected
  line L1989 (184.638, 9.6132) -> (184.638, 3.3431) projected
  line L1990 (184.638, 9.6132) -> (184.638, 3.3431) projected
  line L1991 (184.638, 3.3431) -> (182.914, 3.3431) projected
  line L1992 (184.638, 3.3431) -> (182.914, 3.3431) projected
  line L1993 (182.914, 3.3431) -> (182.914, 2.1429) projected
  line L1994 (182.914, 3.3431) -> (182.914, 2.1429) projected
  line L1995 (179.813, 2.1429) -> (179.813, 3.3431) projected
  line L1996 (179.813, 2.1429) -> (179.813, 3.3431) projected
  line L1997 (179.813, 3.3431) -> (178.088, 3.3431) projected
  line L1998 (179.813, 3.3431) -> (178.088, 3.3431) projected
  line L1999 (182.914, 2.1429) -> (179.813, 2.1429) projected
  line L2000 (182.914, 2.1429) -> (179.813, 2.1429) projected
  line L2001 (193.033, 35.9625) -> (193.033, 22.163) projected
  line L2002 (193.033, 35.9625) -> (193.033, 22.163) projected
  line L2003 (178.088, 12.2136) -> (178.088, 15.4423) projected
  line L2004 (178.088, 15.4423) -> (184.638, 15.4423) projected
  line L2005 (178.088, 12.2136) -> (178.088, 15.4423) projected
  line L2006 (209.702, 3.113) -> (195.902, 3.113) projected
  line L2007 (209.702, 16.9127) -> (209.702, 3.113) projected
  line L2008 (195.902, 16.9127) -> (209.702, 16.9127) projected
  line L2009 (195.902, 16.9127) -> (209.702, 16.9127) projected
  line L2010 (178.088, 15.4423) -> (184.638, 15.4423) projected
  line L2011 (202.558, 41.2129) -> (188.758, 41.2129) projected
  line L2012 (193.033, 35.9625) -> (193.033, 22.163) projected
  line L2013 (179.233, 35.9625) -> (193.033, 35.9625) projected
  line L2014 (193.033, 22.163) -> (179.233, 22.163) projected
  line L2015 (179.233, 35.9625) -> (193.033, 35.9625) projected
  line L2016 (193.033, 35.9625) -> (193.033, 22.163) projected
  line L2017 (193.033, 22.163) -> (179.233, 22.163) projected
  line L2018 (202.558, 41.2129) -> (188.758, 41.2129) projected
  line L2019 (138.264, 12.2136) -> (178.088, 12.2136) projected
  line L2020 (138.264, 12.2136) -> (178.088, 12.2136) projected
  line L2021 (240.658, 55.0125) -> (240.658, 41.2129) projected
  line L2022 (135.883, 35.9625) -> (135.883, 22.163) projected
  line L2023 (135.883, 35.9625) -> (135.883, 22.163) projected
  line L2024 (179.233, 22.163) -> (179.233, 35.9625) projected
  line L2025 (179.233, 22.163) -> (179.233, 35.9625) projected
  line L2026 (160.183, 22.163) -> (160.183, 35.9625) projected
  line L2027 (160.183, 22.163) -> (160.183, 35.9625) projected
  line L2028 (154.933, 35.9625) -> (154.933, 22.163) projected
  line L2029 (154.933, 35.9625) -> (154.933, 22.163) projected
  line L2030 (164.458, 41.2129) -> (150.658, 41.2129) projected
  line L2031 (164.458, 41.2129) -> (150.658, 41.2129) projected
  line L2032 (138.264, 12.2136) -> (178.088, 12.2136) projected
  line L2033 (138.264, 12.2136) -> (178.088, 12.2136) projected
  line L2034 (178.088, 7.8135) -> (138.264, 7.8135) projected
  line L2035 (178.088, 7.8135) -> (138.264, 7.8135) projected
  line L2036 (138.264, 7.8135) -> (138.264, 3.113) projected
  line L2037 (138.264, 7.8135) -> (138.264, 3.113) projected
  line L2038 (154.933, 22.163) -> (141.133, 22.163) projected
  line L2039 (154.933, 22.163) -> (141.133, 22.163) projected
  line L2040 (154.933, 22.163) -> (141.133, 22.163) projected
  line L2041 (154.933, 22.163) -> (141.133, 22.163) projected
  line L2042 (141.133, 22.163) -> (141.133, 35.9625) projected
  line L2043 (141.133, 22.163) -> (141.133, 35.9625) projected
  line L2044 (141.133, 22.163) -> (141.133, 35.9625) projected
  line L2045 (141.133, 22.163) -> (141.133, 35.9625) projected
  line L2046 (141.133, 35.9625) -> (154.933, 35.9625) projected
  line L2047 (141.133, 35.9625) -> (154.933, 35.9625) projected
  line L2048 (141.133, 35.9625) -> (154.933, 35.9625) projected
  line L2049 (141.133, 35.9625) -> (154.933, 35.9625) projected
  line L2050 (145.408, 41.2129) -> (131.608, 41.2129) projected
  line L2051 (145.408, 41.2129) -> (131.608, 41.2129) projected
  line L2052 (154.933, 35.9625) -> (154.933, 22.163) projected
  line L2053 (154.933, 35.9625) -> (154.933, 22.163) projected
  line L2054 (160.183, 22.163) -> (160.183, 35.9625) projected
  line L2055 (160.183, 22.163) -> (160.183, 35.9625) projected
  line L2056 (160.183, 35.9625) -> (173.983, 35.9625) projected
  line L2057 (160.183, 35.9625) -> (173.983, 35.9625) projected
  line L2058 (173.983, 35.9625) -> (173.983, 22.163) projected
  line L2059 (173.983, 35.9625) -> (173.983, 22.163) projected
  line L2060 (173.983, 35.9625) -> (173.983, 22.163) projected
  line L2061 (173.983, 35.9625) -> (173.983, 22.163) projected
  line L2062 (160.183, 35.9625) -> (173.983, 35.9625) projected
  line L2063 (160.183, 35.9625) -> (173.983, 35.9625) projected
  line L2064 (173.983, 22.163) -> (160.183, 22.163) projected
  line L2065 (173.983, 22.163) -> (160.183, 22.163) projected
  line L2066 (173.983, 22.163) -> (160.183, 22.163) projected
  line L2067 (173.983, 22.163) -> (160.183, 22.163) projected
  line L2068 (145.408, 55.0125) -> (145.408, 41.2129) projected
  line L2069 (145.408, 55.0125) -> (145.408, 41.2129) projected
  line L2070 (150.658, 41.2129) -> (150.658, 55.0125) projected
  line L2071 (150.658, 41.2129) -> (150.658, 55.0125) projected
  line L2072 (183.508, 41.2129) -> (169.708, 41.2129) projected
  line L2073 (183.508, 41.2129) -> (169.708, 41.2129) projected
  line L2074 (164.458, 55.0125) -> (164.458, 41.2129) projected
  line L2075 (164.458, 55.0125) -> (164.458, 41.2129) projected
  line L2076 (169.708, 41.2129) -> (169.708, 55.0125) projected
  line L2077 (169.708, 41.2129) -> (169.708, 55.0125) projected
  line L2078 (183.508, 55.0125) -> (183.508, 41.2129) projected
  line L2079 (183.508, 55.0125) -> (183.508, 41.2129) projected
  line L2080 (131.12, 79.3129) -> (117.321, 79.3129) projected
  line L2081 (131.12, 79.3129) -> (117.321, 79.3129) projected
  line L2082 (117.321, 79.3129) -> (117.321, 93.1125) projected
  line L2083 (117.321, 79.3129) -> (117.321, 93.1125) projected
  line L2084 (117.321, 93.1125) -> (131.12, 93.1125) projected
  line L2085 (131.12, 93.1125) -> (131.12, 79.3129) projected
  line L2086 (131.12, 93.1125) -> (131.12, 79.3129) projected
  line L2087 (131.12, 79.3129) -> (117.321, 79.3129) projected
  line L2088 (131.12, 79.3129) -> (117.321, 79.3129) projected
  line L2089 (131.12, 93.1125) -> (131.12, 79.3129) projected
  line L2090 (131.12, 93.1125) -> (131.12, 79.3129) projected
  line L2091 (112.07, 103.125) -> (98.2694, 103.125) projected
  line L2092 (112.07, 103.125) -> (98.2694, 103.125) projected
  line L2093 (117.321, 79.3129) -> (117.321, 93.1125) projected
  line L2094 (117.321, 79.3129) -> (117.321, 93.1125) projected
  line L2095 (112.07, 93.1125) -> (112.07, 79.3129) projected
  line L2096 (112.07, 93.1125) -> (112.07, 79.3129) projected
  line L2097 (112.07, 93.1125) -> (112.07, 79.3129) projected
  line L2098 (98.2694, 93.1125) -> (112.07, 93.1125) projected
  line L2099 (98.2694, 93.1125) -> (112.07, 93.1125) projected
  line L2100 (98.2694, 93.1125) -> (112.07, 93.1125) projected
  line L2101 (98.2694, 93.1125) -> (112.07, 93.1125) projected
  line L2102 (112.07, 79.3129) -> (98.2694, 79.3129) projected
  line L2103 (98.2694, 79.3129) -> (98.2694, 93.1125) projected
  line L2104 (112.07, 79.3129) -> (98.2694, 79.3129) projected
  line L2105 (112.07, 79.3129) -> (98.2694, 79.3129) projected
  line L2106 (98.2694, 79.3129) -> (98.2694, 93.1125) projected
  line L2107 (98.2694, 79.3129) -> (98.2694, 93.1125) projected
  line L2108 (112.07, 79.3129) -> (98.2694, 79.3129) projected
  line L2109 (98.2694, 79.3129) -> (98.2694, 93.1125) projected
  line L2110 (112.07, 93.1125) -> (112.07, 79.3129) projected
  line L2111 (98.2694, 103.125) -> (98.2694, 116.926) projected
  line L2112 (98.2694, 103.125) -> (98.2694, 116.926) projected
  line L2113 (98.2694, 116.926) -> (112.07, 116.926) projected
  line L2114 (98.2694, 116.926) -> (112.07, 116.926) projected
  line L2115 (117.321, 93.1125) -> (131.12, 93.1125) projected
  line L2116 (117.321, 93.1125) -> (131.12, 93.1125) projected
  line L2117 (112.07, 116.926) -> (112.07, 103.125) projected
  line L2118 (112.07, 116.926) -> (112.07, 103.125) projected
  line L2119 (135.883, 103.125) -> (122.083, 103.125) projected
  line L2120 (135.883, 103.125) -> (122.083, 103.125) projected
  line L2121 (122.083, 103.125) -> (122.083, 116.926) projected
  line L2122 (122.083, 103.125) -> (122.083, 116.926) projected
  line L2123 (135.883, 116.926) -> (135.883, 103.125) projected
  line L2124 (135.883, 116.926) -> (135.883, 103.125) projected
  line L2125 (122.083, 116.926) -> (135.883, 116.926) projected
  line L2126 (122.083, 116.926) -> (135.883, 116.926) projected
  line L2127 (117.321, 93.1125) -> (131.12, 93.1125) projected
  line L2128 (185.463, 12.2136) -> (185.463, 9.6132) projected
  line L2129 (185.463, 12.2136) -> (185.463, 9.6132) projected
  line L2130 (184.638, 15.4423) -> (184.638, 12.2136) projected
  line L2131 (184.638, 12.2136) -> (185.463, 12.2136) projected
  line L2132 (184.638, 12.2136) -> (185.463, 12.2136) projected
  line L2133 (184.638, 15.4423) -> (184.638, 12.2136) projected
  line L2134 (185.463, 9.6132) -> (184.638, 9.6132) projected
  line L2135 (185.463, 9.6132) -> (184.638, 9.6132) projected
  line L2136 (184.638, 9.6132) -> (184.638, 3.3431) projected
  line L2137 (184.638, 9.6132) -> (184.638, 3.3431) projected
  line L2138 (184.638, 3.3431) -> (182.914, 3.3431) projected
  line L2139 (184.638, 3.3431) -> (182.914, 3.3431) projected
  line L2140 (182.914, 3.3431) -> (182.914, 2.1429) projected
  line L2141 (182.914, 3.3431) -> (182.914, 2.1429) projected
  line L2142 (182.914, 2.1429) -> (179.813, 2.1429) projected
  line L2143 (182.914, 2.1429) -> (179.813, 2.1429) projected
  line L2144 (179.813, 2.1429) -> (179.813, 3.3431) projected
  line L2145 (179.813, 2.1429) -> (179.813, 3.3431) projected
  line L2146 (179.813, 3.3431) -> (178.088, 3.3431) projected
  line L2147 (179.813, 3.3431) -> (178.088, 3.3431) projected
  line L2148 (178.088, 3.3431) -> (178.088, 7.8135) projected
  line L2149 (178.088, 3.3431) -> (178.088, 7.8135) projected
  line L2150 (178.088, 7.8135) -> (138.264, 7.8135) projected
  line L2151 (178.088, 7.8135) -> (138.264, 7.8135) projected
  line L2152 (178.088, 12.2136) -> (178.088, 15.4423) projected
  line L2153 (178.088, 12.2136) -> (178.088, 15.4423) projected
  line L2154 (178.088, 3.3431) -> (178.088, 7.8135) projected
  line L2155 (178.088, 3.3431) -> (178.088, 7.8135) projected
  line L2156 (140.645, 74.0625) -> (140.645, 60.2629) projected
  line L2157 (140.645, 74.0625) -> (140.645, 60.2629) projected
  line L2158 (140.645, 60.2629) -> (126.846, 60.2629) projected
  line L2159 (140.645, 60.2629) -> (126.846, 60.2629) projected
  line L2160 (126.846, 60.2629) -> (126.846, 74.0625) projected
  line L2161 (126.846, 60.2629) -> (126.846, 74.0625) projected
  line L2162 (126.846, 74.0625) -> (140.645, 74.0625) projected
  line L2163 (126.846, 74.0625) -> (140.645, 74.0625) projected
  line L2164 (145.896, 74.0625) -> (159.695, 74.0625) projected
  line L2165 (145.896, 74.0625) -> (159.695, 74.0625) projected
  line L2166 (159.695, 74.0625) -> (159.695, 60.2629) projected
  line L2167 (159.695, 74.0625) -> (159.695, 60.2629) projected
  line L2168 (159.695, 60.2629) -> (145.896, 60.2629) projected
  line L2169 (159.695, 60.2629) -> (145.896, 60.2629) projected
  line L2170 (145.896, 60.2629) -> (145.896, 74.0625) projected
  line L2171 (145.896, 60.2629) -> (145.896, 74.0625) projected
  line L2172 (131.608, 55.0125) -> (145.408, 55.0125) projected
  line L2173 (131.608, 55.0125) -> (145.408, 55.0125) projected
  line L2174 (145.896, 60.2629) -> (145.896, 74.0625) projected
  line L2175 (145.896, 60.2629) -> (145.896, 74.0625) projected
  line L2176 (140.645, 74.0625) -> (140.645, 60.2629) projected
  line L2177 (140.645, 74.0625) -> (140.645, 60.2629) projected
  line L2178 (126.846, 60.2629) -> (126.846, 74.0625) projected
  line L2179 (126.846, 60.2629) -> (126.846, 74.0625) projected
  line L2180 (140.645, 60.2629) -> (126.846, 60.2629) projected
  line L2181 (140.645, 60.2629) -> (126.846, 60.2629) projected
  line L2182 (126.846, 74.0625) -> (140.645, 74.0625) projected
  line L2183 (126.846, 74.0625) -> (140.645, 74.0625) projected
  line L2184 (150.17, 79.3129) -> (136.371, 79.3129) projected
  line L2185 (150.17, 79.3129) -> (136.371, 79.3129) projected
  line L2186 (124.463, 12.2136) -> (124.463, 16.9127) projected
  line L2187 (124.463, 12.2136) -> (124.463, 16.9127) projected
  line L2188 (122.083, 116.926) -> (135.883, 116.926) projected
  line L2189 (122.083, 116.926) -> (135.883, 116.926) projected
  line L2190 (122.083, 103.125) -> (122.083, 116.926) projected
  line L2191 (122.083, 103.125) -> (122.083, 116.926) projected
  line L2192 (122.083, 35.9625) -> (135.883, 35.9625) projected
  line L2193 (122.083, 35.9625) -> (135.883, 35.9625) projected
  line L2194 (135.883, 22.163) -> (122.083, 22.163) projected
  line L2195 (135.883, 22.163) -> (122.083, 22.163) projected
  line L2196 (122.083, 22.163) -> (122.083, 35.9625) projected
  line L2197 (122.083, 22.163) -> (122.083, 35.9625) projected
  line L2198 (124.463, 16.9127) -> (138.264, 16.9127) projected
  line L2199 (124.463, 16.9127) -> (138.264, 16.9127) projected
  line L2200 (138.264, 16.9127) -> (138.264, 12.2136) projected
  line L2201 (138.264, 16.9127) -> (138.264, 12.2136) projected
  line L2202 (138.264, 7.8135) -> (138.264, 3.113) projected
  line L2203 (138.264, 7.8135) -> (138.264, 3.113) projected
  line L2204 (138.264, 3.113) -> (124.463, 3.113) projected
  line L2205 (138.264, 3.113) -> (124.463, 3.113) projected
  line L2206 (124.463, 3.113) -> (124.463, 7.8135) projected
  line L2207 (124.463, 3.113) -> (124.463, 7.8135) projected
  line L2208 (122.083, 35.9625) -> (135.883, 35.9625) projected
  line L2209 (122.083, 35.9625) -> (135.883, 35.9625) projected
  line L2210 (135.883, 35.9625) -> (135.883, 22.163) projected
  line L2211 (135.883, 35.9625) -> (135.883, 22.163) projected
  line L2212 (135.883, 22.163) -> (122.083, 22.163) projected
  line L2213 (135.883, 22.163) -> (122.083, 22.163) projected
  line L2214 (124.463, 12.2136) -> (124.463, 16.9127) projected
  line L2215 (124.463, 12.2136) -> (124.463, 16.9127) projected
  line L2216 (124.463, 3.113) -> (124.463, 7.8135) projected
  line L2217 (124.463, 3.113) -> (124.463, 7.8135) projected
  line L2218 (138.264, 3.113) -> (124.463, 3.113) projected
  line L2219 (138.264, 3.113) -> (124.463, 3.113) projected
  line L2220 (138.264, 16.9127) -> (138.264, 12.2136) projected
  line L2221 (138.264, 16.9127) -> (138.264, 12.2136) projected
  line L2222 (124.463, 16.9127) -> (138.264, 16.9127) projected
  line L2223 (124.463, 16.9127) -> (138.264, 16.9127) projected
  line L2224 (116.833, 35.9625) -> (116.833, 22.163) projected
  line L2225 (116.833, 35.9625) -> (116.833, 22.163) projected
  line L2226 (112.558, 41.2129) -> (112.558, 55.0125) projected
  line L2227 (112.558, 41.2129) -> (112.558, 55.0125) projected
  line L2228 (112.558, 55.0125) -> (126.358, 55.0125) projected
  line L2229 (112.558, 55.0125) -> (126.358, 55.0125) projected
  line L2230 (126.358, 55.0125) -> (126.358, 41.2129) projected
  line L2231 (126.358, 55.0125) -> (126.358, 41.2129) projected
  line L2232 (112.558, 41.2129) -> (112.558, 55.0125) projected
  line L2233 (112.558, 41.2129) -> (112.558, 55.0125) projected
  line L2234 (103.033, 35.9625) -> (116.833, 35.9625) projected
  line L2235 (103.033, 35.9625) -> (116.833, 35.9625) projected
  line L2236 (103.033, 35.9625) -> (116.833, 35.9625) projected
  line L2237 (103.033, 35.9625) -> (116.833, 35.9625) projected
  line L2238 (126.358, 41.2129) -> (112.558, 41.2129) projected
  line L2239 (126.358, 41.2129) -> (112.558, 41.2129) projected
  line L2240 (126.358, 41.2129) -> (112.558, 41.2129) projected
  line L2241 (126.358, 41.2129) -> (112.558, 41.2129) projected
  line L2242 (126.358, 55.0125) -> (126.358, 41.2129) projected
  line L2243 (126.358, 55.0125) -> (126.358, 41.2129) projected
  line L2244 (112.558, 55.0125) -> (126.358, 55.0125) projected
  line L2245 (112.558, 55.0125) -> (126.358, 55.0125) projected
  line L2246 (131.608, 41.2129) -> (131.608, 55.0125) projected
  line L2247 (131.608, 41.2129) -> (131.608, 55.0125) projected
  line L2248 (107.308, 55.0125) -> (107.308, 41.2129) projected
  line L2249 (103.033, 22.163) -> (103.033, 35.9625) projected
  line L2250 (103.033, 22.163) -> (103.033, 35.9625) projected
  line L2251 (116.833, 35.9625) -> (116.833, 22.163) projected
  line L2252 (116.833, 35.9625) -> (116.833, 22.163) projected
  line L2253 (116.833, 22.163) -> (103.033, 22.163) projected
  line L2254 (97.7829, 35.9625) -> (97.7829, 22.163) projected
  line L2255 (97.7829, 35.9625) -> (97.7829, 22.163) projected
  line L2256 (83.9833, 22.163) -> (83.9833, 35.9625) projected
  line L2257 (83.9833, 22.163) -> (83.9833, 35.9625) projected
  line L2258 (97.7829, 35.9625) -> (97.7829, 22.163) projected
  line L2259 (97.7829, 35.9625) -> (97.7829, 22.163) projected
  line L2260 (103.033, 22.163) -> (103.033, 35.9625) projected
  line L2261 (103.033, 22.163) -> (103.033, 35.9625) projected
  line L2262 (122.083, 22.163) -> (122.083, 35.9625) projected
  line L2263 (122.083, 22.163) -> (122.083, 35.9625) projected
  line L2264 (78.7329, 35.9625) -> (78.7329, 22.163) projected
  line L2265 (78.7329, 35.9625) -> (78.7329, 22.163) projected
  line L2266 (97.7829, 22.163) -> (83.9833, 22.163) projected
  line L2267 (97.7829, 22.163) -> (83.9833, 22.163) projected
  line L2268 (97.7829, 22.163) -> (83.9833, 22.163) projected
  line L2269 (97.7829, 22.163) -> (83.9833, 22.163) projected
  line L2270 (116.833, 22.163) -> (103.033, 22.163) projected
  line L2271 (116.833, 22.163) -> (103.033, 22.163) projected
  line L2272 (116.833, 22.163) -> (103.033, 22.163) projected
  line L2273 (84.6391, 12.2136) -> (124.463, 12.2136) projected
  line L2274 (84.6391, 12.2136) -> (124.463, 12.2136) projected
  line L2275 (84.6391, 12.2136) -> (124.463, 12.2136) projected
  line L2276 (124.463, 7.8135) -> (84.6391, 7.8135) projected
  line L2277 (124.463, 7.8135) -> (84.6391, 7.8135) projected
  line L2278 (124.463, 7.8135) -> (84.6391, 7.8135) projected
  line L2279 (124.463, 7.8135) -> (84.6391, 7.8135) projected
  line L2280 (84.6391, 12.2136) -> (124.463, 12.2136) projected
  line L2281 (107.308, 55.0125) -> (107.308, 41.2129) projected
  line L2282 (107.308, 41.2129) -> (93.5083, 41.2129) projected
  line L2283 (93.5083, 41.2129) -> (93.5083, 55.0125) projected
  line L2284 (93.5083, 55.0125) -> (107.308, 55.0125) projected
  line L2285 (107.308, 41.2129) -> (93.5083, 41.2129) projected
  line L2286 (93.5083, 41.2129) -> (93.5083, 55.0125) projected
  line L2287 (93.5083, 55.0125) -> (107.308, 55.0125) projected
  line L2288 (107.308, 41.2129) -> (93.5083, 41.2129) projected
  line L2289 (107.308, 41.2129) -> (93.5083, 41.2129) projected
  line L2290 (93.5083, 55.0125) -> (107.308, 55.0125) projected
  line L2291 (93.5083, 55.0125) -> (107.308, 55.0125) projected
  line L2292 (83.9833, 35.9625) -> (97.7829, 35.9625) projected
  line L2293 (83.9833, 35.9625) -> (97.7829, 35.9625) projected
  line L2294 (83.9833, 35.9625) -> (97.7829, 35.9625) projected
  line L2295 (83.9833, 35.9625) -> (97.7829, 35.9625) projected
  line L2296 (107.308, 55.0125) -> (107.308, 41.2129) projected
  line L2297 (107.308, 55.0125) -> (107.308, 41.2129) projected
  line L2298 (102.545, 74.0625) -> (102.545, 60.2629) projected
  line L2299 (102.545, 74.0625) -> (102.545, 60.2629) projected
  line L2300 (102.545, 60.2629) -> (88.7444, 60.2629) projected
  line L2301 (102.545, 60.2629) -> (88.7444, 60.2629) projected
  line L2302 (88.7444, 74.0625) -> (102.545, 74.0625) projected
  line L2303 (88.7444, 74.0625) -> (102.545, 74.0625) projected
  line L2304 (107.794, 60.2629) -> (107.794, 74.0625) projected
  line L2305 (107.794, 60.2629) -> (107.794, 74.0625) projected
  line L2306 (107.794, 74.0625) -> (121.595, 74.0625) projected
  line L2307 (107.794, 74.0625) -> (121.595, 74.0625) projected